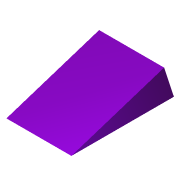
# Autodesk Inventor part: Goal Guide 2
Saved by Autodesk Inventor 2015 SP1 (Build 190203100, 203)
## iProperties
Created: 2014-09-14
Part Number: Goal Guide 2
Document SubType Name: Modeling
Designer: Family Room
Density: 1 g/cm^3
Material: Generic
Appearance: Smooth - Purple
Author: Family Room
Autodesk Inventor part; units mm, degrees
ref_plane "YZ Plane" through (0, 0, 0) normal (1, 0, 0) x (0, 1, 0)
ref_plane "XZ Plane" through (0, 0, 0) normal (0, 1, 0) x (-1, 0, 0)
ref_plane "XY Plane" through (0, 0, 0) normal (0, 0, 1) x (1, 0, 0)
sketch "Sketch1" plane through (0, 0, 0) normal (0, 0, 1) x (1, 0, 0)
  line L0 (0, 0) -> (50.8, 0)
  line L1 (50.8, 0) -> (50.8, 50.8)
  line L2 (50.8, 50.8) -> (0, 50.8)
  line L3 (0, 50.8) -> (0, 0)
  dimension "d0" = 50.8
  dimension "d1" = 50.8
  constraints: 8 end point, 2 parallel, 1 horizontal, 1 perpendicular
  measures "d0" distance of L2.end L1.end
  measures "d1" distance of L1.end L0.end
extrude "Extrusion1" add sketch "Sketch1" along normal blind 127
sketch "Sketch2" plane through (50.8, 0, 0) normal (1, 0, 0) x (0, 0, -1)
  line L0 (-127, 50.8) -> (-127, 0) projected
  line L1 (0, 0) -> (-127, 0) projected
  line L2 (0, 0) -> (0, 50.8) projected
  line L3 (0, 50.8) -> (-127, 50.8) projected
  line L4 (-127, 0) -> (-66.6079, 19.6226)
  line L5 (-127, 0) -> (-63.5, 0) construction
  line L6 (-66.6079, 19.6226) -> (-60.2321, 0)
  line L7 (-60.2321, 0) -> (-127, 0)
  dimension "d4" = 63.5
  dimension "d5" = 18
  constraints: 8 end point, 1 collinear, 1 equal length, 1 horizontal, 1 perpendicular, 1 point on line
  measures "d4" distance of L0.end L4.end
  measures "d5" angle of L5 L4
extrude "Extrusion2" cut sketch "Sketch2" against normal blind 127 contours L3 L2 L1 L6 L4 L0
sketch "Sketch3" plane through (50.8, 0, 127) normal (1, 0, 0) x (0, 0, -1)
  line L0 (66.7679, 0) -> (60.3921, 19.6226) projected
  line L1 (60.3921, 19.6226) -> (0, 0) projected
  line L2 (66.7679, 0) -> (0, 0) projected
  line L3 (60.3921, 19.6226) -> (-12.0784, -3.9245)
  line L4 (-12.0784, -3.9245) -> (70.1883, -3.9245)
  line L5 (60.3921, 19.6226) -> (68.043, -3.9245)
  point P0 (127, 0)
  dimension "d8" = 76.2
  constraints: 6 end point, 1 collinear, 1 parallel, 1 perpendicular, 1 point on line
  measures "d8" distance of L0.end L3.end
extrude "Extrusion3" add sketch "Sketch3" against normal blind 50.8 contours L5 L4 L3 L2
body "Solid1"
